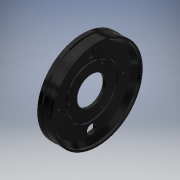
# Autodesk Inventor part: Disc
Saved by Autodesk Inventor 2017 (Build 210142000, 142)
## iProperties
Created: 2016-04-18
Part Number: Disc
Material: Acetal Resin, Black
Document SubType Name: Modeling
Designer: jbreeden
Density: 1.425 g/cm^3
Appearance: Smooth - Black
Mass: 88.1058 g
Surface Area: 334.213 cm^2
Volume: 61.8286 cm^3
Author: jbreeden
Autodesk Inventor part; units mm, degrees
ref_plane "YZ Plane" through (0, 0, 0) normal (1, 0, 0) x (0, 1, 0)
ref_plane "XZ Plane" through (0, 0, 0) normal (0, 1, 0) x (-1, 0, 0)
ref_plane "XY Plane" through (0, 0, 0) normal (0, 0, 1) x (1, 0, 0)
sketch "Sketch1" plane through (0, 0, 0) normal (0, 0, 1) x (1, 0, 0)
  line L0 (0, 0) -> (-10.033, 0)
  line L1 (-10.033, 0) -> (-10.033, -60.198)
  line L2 (-10.033, -60.198) -> (-4.953, -60.198)
  line L3 (-4.953, -60.198) -> (-4.953, -59.182)
  line L4 (-4.953, -59.182) -> (4.953, -59.182)
  line L5 (4.953, -59.182) -> (4.953, -60.198)
  line L6 (4.953, -60.198) -> (10.033, -60.198)
  line L7 (10.033, -60.198) -> (10.033, -57.658)
  line L8 (10.033, -57.658) -> (-10.033, -57.658)
  dimension "d0" = 10.033
  dimension "d1" = 60.198
  dimension "d2" = 5.08
  dimension "d3" = 1.016
  dimension "d4" = 9.906
  dimension "d5" = 1.016
  dimension "d6" = 5.08
  dimension "d7" = 2.54
  constraints: 18 end point, 5 perpendicular, 3 point on line, 1 horizontal, 1 vertical
  measures "d0" distance of L0.start L0.end
  measures "d1" distance of L0.end L1.end
  measures "d2" distance of L1.end L2.end
  measures "d3" distance of L2.end L3.end
  measures "d4" distance of L3.end L4.end
  measures "d5" distance of L4.end L5.end
  measures "d6" distance of L5.end L6.end
  measures "d7" distance of L6.end L7.end
revolve "Revolution1" add sketch "Sketch1" angle 360 about axis through (0, 0, 0) along (-1, 0, 0)
chamfer "Chamfer1" distance 1.016 angle 45 2 edges at (-4.953, 59.182, 0) (4.953, 59.182, 0)
sketch "Sketch2" plane through (0, 0, 0) normal (1, 0, 0) x (0, 1, 0)
  circle A0 centre (0, 0) radius 59.182
  circle A1 centre (0, 0) radius 19.05
  dimension "d12" = 118.364
  dimension "d13" = 38.1
  constraints: 2 centre point, 2 coincident
  measures "d12" diameter of A0
  measures "d13" diameter of A1
extrude "Extrusion1" add sketch "Sketch2" along normal mid plane 3.81
chamfer "Chamfer2" distance 5.08 angle 45 2 edges at (1.905, 57.658, 0) (-1.905, 57.658, 0)
sketch "Sketch3" plane through (1.905, 0, 0) normal (1, 0, 0) x (0, 0, -1)
  line L0 (0, 0) -> (-29.3624, 0)
  dimension "d19" = 29.3624
  constraints: 2 end point, 1 horizontal
  measures "d19" distance of L0.start L0.end
hole "Hole1" at (1.905, 0, 29.3624) direction (-1, 0, 0) diameter 3.5052 end through all
pattern_circular "Circular Pattern1" count 3 over 360 about axis through (0, 0, 0) along (1, 0, 0) of "Hole1"
sketch "Sketch4" plane through (1.905, 0, 0) normal (1, 0, 0) x (0, 0, -1)
  circle A0 centre (0, 0) radius 32.385
  circle A1 centre (0, 0) radius 35.4838
  dimension "d30" = 64.77
  dimension "d31" = 70.9676
  constraints: 2 centre point, 2 coincident
  measures "d30" diameter of A0
  measures "d31" diameter of A1
extrude "Extrusion2" cut sketch "Sketch4" against normal blind 1.8796
sketch "Sketch5" plane through (1.905, 0, 0) normal (1, 0, 0) x (0, 0, -1)
  line L0 (0, 0) -> (43.18, 0)
  line L1 (0, 0) -> (0, 25.4)
  line L2 (0, 0) -> (-43.18, 0)
  dimension "d34" = 43.18
  dimension "d35" = 25.4
  constraints: 6 end point, 1 horizontal, 1 symmetric about line, 1 vertical
  measures "d34" distance of L0.start L0.end
  measures "d35" distance of L0.start L1.end
hole "Hole2" at (1.905, 0, 43.18) at (1.905, 0, -43.18) direction (-1, 0, 0) diameter 4.064 end through all
sketch "Sketch6" plane through (1.905, 0, 0) normal (1, 0, 0) x (0, 0, -1)
  circle A0 centre (0, 0) radius 36.195
  line L0 (0, 36.195) -> (0, 37.465)
  line L1 (0, 37.465) -> (-3.175, 37.465)
  line L2 (-3.175, 37.465) -> (3.175, 37.465)
  line L3 (3.175, 37.465) -> (3.175, 50.165)
  line L4 (3.175, 50.165) -> (-3.175, 50.165)
  line L5 (-3.175, 50.165) -> (-3.175, 37.465)
  dimension "d43" = 72.39
  dimension "d44" = 1.27
  dimension "d45" = 3.175
  dimension "d46" = 6.35
  dimension "d47" = 12.7
  constraints: 12 end point, 2 parallel, 2 perpendicular, 1 coincident, 1 horizontal, 1 vertical, 1 vertical alignment, 2 other
  measures "d44" distance of L0.start L0.end
  measures "d45" distance of L0.end L1.end
  measures "d46" distance of L4.end L3.end
  measures "d47" distance of L3.end L2.end
extrude "Extrusion3" cut sketch "Sketch6" against normal blind 1.778 contours L1 L5 L4 L3 L2
sketch "Sketch7" plane through (0.127, 0, 0) normal (1, 0, 0) x (0, 0, -1)
  line L0 (3.175, 37.465) -> (-3.175, 37.465) projected
  line L1 (-3.175, 37.465) -> (-1.27, 37.465)
  line L2 (-1.27, 37.465) -> (-1.27, 38.735)
  line L3 (-1.27, 38.735) -> (-1.27, 41.275)
  line L4 (-1.27, 41.275) -> (-1.27, 43.815)
  line L5 (-1.27, 43.815) -> (-1.27, 46.355)
  line L6 (-1.27, 46.355) -> (-1.27, 48.895)
  line L7 (0, 37.465) -> (0, 50.165)
  line L8 (-3.175, 50.165) -> (3.175, 50.165) projected
  line L9 (1.27, 37.465) -> (1.27, 38.735)
  line L10 (1.27, 38.735) -> (1.27, 41.275)
  line L11 (1.27, 41.275) -> (1.27, 43.815)
  line L12 (1.27, 43.815) -> (1.27, 46.355)
  line L13 (1.27, 46.355) -> (1.27, 48.895)
  point P0 (0, 0)
  dimension "d50" = 1.905
  dimension "d51" = 1.27
  dimension "d52" = 2.54
  dimension "d53" = 2.54
  dimension "d54" = 2.54
  dimension "d55" = 2.54
  dimension "d56" = 12.7
  constraints: 24 end point, 7 point on line, 6 symmetric about line, 2 midpoint, 1 perpendicular, 1 vertical
  measures "d50" distance of L0.end L1.end
  measures "d51" distance of L1.end L2.end
  measures "d52" distance of L2.end L3.end
  measures "d53" distance of L3.end L4.end
  measures "d54" distance of L4.end L5.end
  measures "d55" distance of L5.end L6.end
  measures "d56" distance of L7.start L7.end
hole "Hole3" at (0.127, 48.895, 1.27) at (0.127, 46.355, 1.27) at (0.127, 43.815, 1.27) at (0.127, 41.275, 1.27) at (0.127, 38.735, 1.27) at (0.127, 38.735, -1.27) at (0.127, 41.275, -1.27) at (0.127, 43.815, -1.27) at (0.127, 46.355, -1.27) at (0.127, 48.895, -1.27) direction (-1, 0, 0) diameter 1.27 end through all
fillet "Fillet1" radius 3.175 4 edges at (1.016, 37.465, -3.175) (1.016, 50.165, -3.175) (1.016, 50.165, 3.175) (1.016, 37.465, 3.175)
sketch "Sketch8" plane through (1.905, 0, 0) normal (1, 0, 0) x (0, 0, -1)
  circle A0 centre (0, -44.45) radius 6.1516
  point P0 (0, 0)
  dimension "d65" = 12.3031
  dimension "d66" = 44.45
  constraints: 1 centre point
  measures "d65" diameter of A0
  measures "d66" distance of point (0, 0) A0.centre
extrude "Extrusion4" cut sketch "Sketch8" against normal blind 25.4
body "Solid1"
